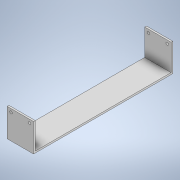
# Autodesk Inventor part: LiftBrace
Saved by Autodesk Inventor 2020 (Build 240168000, 168)
## iProperties
Created: 2020-01-19
Part Number: LiftBrace
Material: Generic
Document SubType Name: Modeling
Designer: tdmp4
Density: 1 g/cm^3
Appearance: Default
Author: tdmp4
Autodesk Inventor part; units mm, degrees
ref_plane "YZ Plane" through (0, 0, 0) normal (1, 0, 0) x (0, 1, 0)
ref_plane "XZ Plane" through (0, 0, 0) normal (0, 1, 0) x (-1, 0, 0)
ref_plane "XY Plane" through (0, 0, 0) normal (0, 0, 1) x (1, 0, 0)
sketch "Sketch1" plane through (0, 0, 0) normal (0, 1, 0) x (-1, 0, 0)
  line L0 (0, 0) -> (38.1, 0)
  line L1 (38.1, 0) -> (38.1, -201.295)
  line L2 (38.1, -201.295) -> (0, -201.295)
  line L3 (0, -201.295) -> (0, 0)
  dimension "d0" = 201.295
  dimension "d1" = 38.1
  constraints: 8 end point, 2 parallel, 1 horizontal, 1 perpendicular
  measures "d0" distance of L2.end L0.start
  measures "d1" distance of L0.start L0.end
extrude "Extrusion1" add sketch "Sketch1" along normal blind 2.54
sketch "Sketch2" plane through (0, 2.54, 0) normal (0, 1, 0) x (1, 0, 0)
  line L0 (-38.1, 201.295) -> (-38.1, 0) projected
  line L1 (-38.1, 0) -> (0, 0) projected
  line L2 (0, 0) -> (0, 201.295) projected
  line L3 (-38.1, 0) -> (0, 0)
  line L4 (0, 0) -> (0, 2.535)
  line L5 (0, 2.535) -> (-38.1, 2.535)
  line L6 (-38.1, 2.535) -> (-38.1, 0)
  line L7 (0, 201.295) -> (-38.1, 201.295)
  line L8 (-38.1, 201.295) -> (-38.1, 198.7847)
  line L9 (-38.1, 198.7847) -> (0, 198.7847)
  line L10 (0, 198.7847) -> (0, 201.295)
  constraints: 16 end point, 4 parallel, 2 horizontal, 2 perpendicular, 2 point on line
extrude "Extrusion2" add sketch "Sketch2" along normal blind 38.1 contours L7 L2 L9 L0 | L5 L2 L1 L0
sketch "Sketch3" plane through (0, 0, -201.295) normal (0, 0, -1) x (-1, 0, 0)
  line L0 (38.1, 40.64) -> (0, 40.64) projected
  line L1 (19.05, 40.64) -> (19.05, 0)
  line L2 (38.1, 0) -> (0, 0) projected
  line L3 (0, 0) -> (0, 40.64) projected
  line L4 (0, 20.32) -> (38.1, 20.32)
  line L5 (38.1, 2.54) -> (38.1, 40.64) projected
  circle A0 centre (19.05, 35.9001) radius 13.4747
  circle A1 centre (32.5247, 35.9001) radius 1.7907
  circle A2 centre (5.5753, 35.9001) radius 1.7907
  dimension "d11" = 26.9494
  dimension "d12" = 3.5814
  dimension "d13" = 3.5814
  constraints: 4 end point, 3 centre point, 3 midpoint, 2 point on circle, 2 point on line, 1 perpendicular
  measures "d11" diameter of A0
  measures "d12" diameter of A1
  measures "d13" diameter of A2
extrude "Extrusion3" cut sketch "Sketch3" against normal blind 246.0625 contours A1 A0 | A0 A1 | A2 A0 | A0 A2
body "Solid1"
